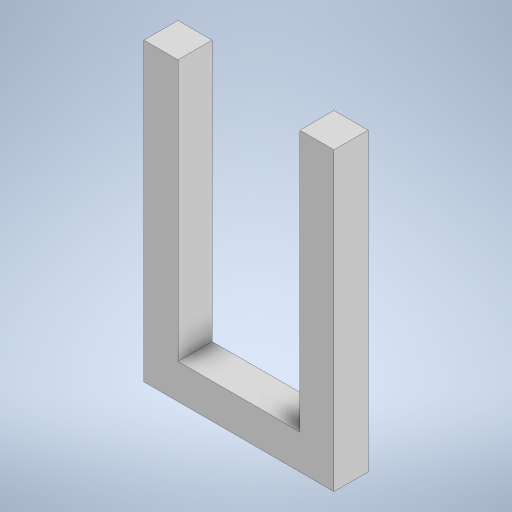
# Autodesk Inventor part: servo-clamp
Saved by Autodesk Inventor 2024 (Build 280153000, 153)
## iProperties
Created: 2024-01-23
Part Number: servo-clamp
Material: Generic
Document SubType Name: Modeling
Designer: emosh
Density: 1 g/cm^3
Appearance: Default
Author: emosh
## iProperties of the stored document servo-clamp_3DPrint.ipt
Created: 2024-01-24
Part Number: servo-clamp_3DPrint
Material: Generic
Document SubType Name: Modeling
Designer: emosh
Density: 1 g/cm^3
Appearance: Default
Author: emosh
Autodesk Inventor part; units mm, degrees
ref_plane "YZ Plane" through (0, 0, 0) normal (1, 0, 0) x (0, 1, 0)
ref_plane "XZ Plane" through (0, 0, 0) normal (0, 1, 0) x (-1, 0, 0)
ref_plane "XY Plane" through (0, 0, 0) normal (0, 0, 1) x (1, 0, 0)
sketch "Sketch1" plane through (0, 0, 0) normal (0, 1, 0) x (-1, 0, 0)
  line L0 (0, 0) -> (22.225, 0)
  line L1 (22.225, 0) -> (22.225, -6.223)
  line L2 (22.225, -6.223) -> (0, -6.223)
  line L3 (0, -6.223) -> (0, 0)
  line L4 (0, 0) -> (-6.223, 0)
  line L5 (-6.223, 0) -> (-6.223, -6.223)
  line L6 (-6.223, -6.223) -> (0, -6.223)
  line L7 (0, -6.223) -> (0, 0)
  line L8 (22.225, 0) -> (28.448, 0)
  line L9 (28.448, 0) -> (28.448, -6.223)
  line L10 (28.448, -6.223) -> (22.225, -6.223)
  line L11 (22.225, -6.223) -> (22.225, 0)
  dimension "d0" = 22.225
  dimension "d1" = 6.223
  dimension "d2" = 6.223
  dimension "d3" = 6.223
  constraints: 24 end point, 6 parallel, 3 horizontal, 3 perpendicular, 2 point on line
  measures "d0" distance of L1.end L2.end
  measures "d1" distance of L0.end L1.end
  measures "d2" distance of L6.end L5.end
  measures "d3" distance of L9.end L10.end
extrude "Extrusion1" add sketch "Sketch1" along normal blind 53.975
sketch "Sketch2" plane through (0, 53.975, 0) normal (0, 1, 0) x (1, 0, 0)
  line L0 (6.223, 6.223) -> (-28.448, 6.223) projected
  line L1 (0, 0) -> (-22.225, 0)
  line L2 (-22.225, 0) -> (-22.225, 6.223)
  line L3 (-22.225, 6.223) -> (0, 6.223)
  line L4 (0, 6.223) -> (0, 0)
  point P0 (0, 6.223)
  dimension "d6" = 22.225
  constraints: 8 end point, 2 parallel, 1 horizontal, 1 perpendicular, 1 point on line
  measures "d6" distance of L2.end L3.end
extrude "Extrusion2" cut sketch "Sketch2" against normal blind 47.625
sketch "Sketch7" plane through (0, 53.975, 0) normal (0, 1, 0) x (1, 0, 0)
  point P0 (0, 0)
body "Solid1"
